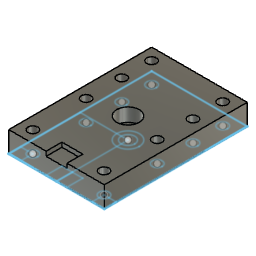
EOM_pcb_adapter v6 (Autodesk Fusion 360 design; units mm, degrees)
Autodesk Fusion 360 part; units mm, degrees
note: some values were not read from the file. Set by a fixed rule: which sketch regions a step uses.
sketch "Sketch1" plane through (0, 0, 0) normal (0, 0, 1) x (1, 0, 0)
  line L0 (8.9904, 12.5053) -> (41.0904, 12.5053)
  line L1 (41.0904, 12.5053) -> (41.0904, 60.5053)
  line L2 (41.0904, 60.5053) -> (8.9904, 60.5053)
  line L3 (8.9904, 60.5053) -> (8.9904, 12.5053)
  line L4 (41.0904, 60.5053) -> (8.9904, 60.5053)
  line L5 (8.9904, 60.5053) -> (8.9904, 12.5053)
  line L6 (8.9904, 12.5053) -> (41.0904, 12.5053)
  line L7 (41.0904, 12.5053) -> (41.0904, 60.5053)
  line L8 (8.9904, 12.5053) -> (41.0904, 12.5053)
  line L9 (41.0904, 12.5053) -> (41.0904, 60.5053)
  line L10 (41.0904, 60.5053) -> (8.9904, 60.5053)
  line L11 (8.9904, 60.5053) -> (8.9904, 12.5053)
  line L12 (8.9904, 12.5053) -> (13.0904, 12.5053)
  line L13 (13.0904, 12.5053) -> (13.0904, 16.5053)
  line L14 (13.0904, 16.5053) -> (8.9904, 16.5053)
  line L15 (8.9904, 16.5053) -> (8.9904, 12.5053)
  line L16 (41.0904, 12.5053) -> (36.9904, 12.5053)
  line L17 (36.9904, 12.5053) -> (36.9904, 16.5053)
  line L18 (36.9904, 16.5053) -> (41.0904, 16.5053)
  line L19 (41.0904, 16.5053) -> (41.0904, 12.5053)
  line L20 (8.9904, 12.5053) -> (25.0404, 12.5053)
  line L21 (25.0404, 12.5053) -> (25.0404, 36.5053)
  line L22 (25.0404, 36.5053) -> (8.9904, 36.5053)
  line L23 (8.9904, 36.5053) -> (8.9904, 12.5053)
  circle A0 centre (25.0404, 36.5053) radius 2.25
  line L24 (25.0404, 12.5053) -> (28.5404, 12.5053)
  line L25 (28.5404, 12.5053) -> (28.5404, 17.8053)
  line L26 (28.5404, 17.8053) -> (25.0404, 17.8053)
  line L27 (25.0404, 17.8053) -> (25.0404, 12.5053)
  line L28 (25.0404, 12.5053) -> (21.5404, 12.5053)
  line L29 (21.5404, 12.5053) -> (21.5404, 17.8053)
  line L30 (21.5404, 17.8053) -> (25.0404, 17.8053)
  line L31 (25.0404, 17.8053) -> (25.0404, 12.5053)
  circle A1 centre (12.9235, 34.5524) radius 1.625
  circle A2 centre (12.9235, 46.5524) radius 1.625
  circle A3 centre (12.9235, 56.5524) radius 1.625
  circle A4 centre (36.8235, 56.5524) radius 1.625
  circle A5 centre (36.8235, 46.5524) radius 1.625
  circle A6 centre (36.8235, 34.5524) radius 1.625
  circle A7 centre (36.9904, 16.5053) radius 1.625
  circle A8 centre (13.0904, 16.5053) radius 1.625
  circle A9 centre (25.0404, 36.5053) radius 3.75
  point P0 (12.9235, 16.5524)
  dimension "d1" = 32.1
  dimension "d2" = 48
  dimension "d5" = 4.1
  dimension "d6" = 4
  dimension "d8" = 4.1
  dimension "d9" = 4
  dimension "d17" = 16.05
  dimension "d18" = 24
  dimension "d20" = 4.5
  dimension "d21" = 3.5
  dimension "d22" = 5.3
  dimension "d23" = 3.5
  dimension "d24" = 5.3
  dimension "d31" = 3.25
  dimension "d32" = 3.25
  dimension "d33" = 3.25
  dimension "d34" = 3.25
  dimension "d35" = 3.25
  dimension "d36" = 3.25
  dimension "d37" = 3.25
  dimension "d38" = 3.25
  dimension "d45" = 7.5
  constraint horizontal L0
  constraint vertical L1
  constraint horizontal L2
  constraint vertical L3
  constraint horizontal L4
  constraint vertical L5
  constraint horizontal L6
  constraint vertical L7
  constraint horizontal L8
  constraint vertical L9
  constraint horizontal L10
  constraint vertical L11
  constraint horizontal L12
  constraint vertical L13
  constraint horizontal L14
  constraint vertical L15
  constraint horizontal L16
  constraint vertical L17
  constraint horizontal L18
  constraint vertical L19
  constraint horizontal L20
  constraint vertical L21
  constraint horizontal L22
  constraint vertical L23
  constraint horizontal L24
  constraint vertical L25
  constraint horizontal L26
  constraint vertical L27
  constraint horizontal L28
  constraint vertical L29
  constraint horizontal L30
  constraint vertical L31
  constraint coincident L17.end L18.start
  constraint concentric A0 A9
  measures "d1" distance of L0.start L0.end
  measures "d2" distance of L0.start L2.end
  measures "d5" distance of L0.start L12.end
  measures "d6" distance of L0.start L14.end
  measures "d8" distance of L0.end L16.end
  measures "d9" distance of L0.end L18.end
  measures "d17" distance of L0.start L20.end
  measures "d18" distance of L0.start L22.end
  measures "d20" diameter of A0
  measures "d21" distance of L20.end L24.end
  measures "d22" distance of L20.end L26.end
  measures "d23" distance of L20.end L28.end
  measures "d24" distance of L20.end L26.end
  measures "d31" diameter of A1
  measures "d32" diameter of A2
  measures "d33" diameter of A3
  measures "d34" diameter of A4
  measures "d35" diameter of A5
  measures "d36" diameter of A6
  measures "d37" diameter of A7
  measures "d38" diameter of A8
  measures "d45" diameter of A9
extrude "Extrude8" add sketch "Sketch1" along normal blind 7 contours L0 L3 L5 L6 L8 L11 L12 L13 L14 L15 L20 L23 A8 | L0 L3 L5 L6 L8 L11 L13 L14 L20 L21 L22 L23 L29 L30 A8 A9 | L0 L1 L2 L3 L4 L5 L6 L7 L8 L9 L10 L11 L17 L18 L21 L22 L25 L26 A7 A9 | L0 L1 L6 L7 L8 L9 L16 L17 L18 L19 A7
extrude "Extrude9" add sketch "Sketch1" along normal blind 5.5 contours L0 L6 L8 L20 L21 L27 L28 L29 L30 L31 | L0 L6 L8 L21 L24 L25 L26 L27 L31
extrude "Extrude10" add sketch "Sketch1" along normal blind 2.5 contours L21 L22 A0 A9 | L21 L22 A0 A9
